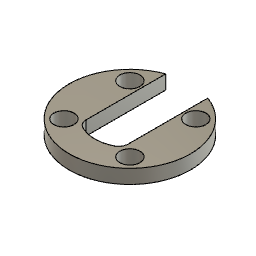
cryo boom 2 v16 (Autodesk Fusion 360 archive; units mm, degrees)
design "cryo clamp lower"
Autodesk Fusion 360 part; units mm, degrees
note: some values were not read from the file. Set by a fixed rule: the direction of a hole.
sketch "Sketch1" plane through (0, 0, 0) normal (0, 1, 0) x (1, 0, 0)
  circle A0 centre (0, 0) radius 13
  circle A1 centre (0, 0) radius 7.5
  line L0 (-4.5, 12.1963) -> (-4.5, -6)
  line L1 (4.5, -6) -> (4.5, 12.1963)
  circle A2 centre (0, 0) radius 10 construction
  line L2 (0, 0) -> (7.0711, -7.0711)
  line L3 (0, 0) -> (13, 0) construction
  point P0 (7.0711, -7.0711)
  dimension "d1" = 26
  dimension "d2" = 15
  dimension "d3" = 9
  dimension "d4" = 20
  dimension "d12" = 45
  constraint coincident A0.centre A1.centre
  constraint coincident A0 L0.start
  constraint coincident A1 L0.end
  constraint vertical L0
  constraint coincident A1 L1.start
  constraint coincident A0 L1.end
  constraint parallel L0 L1
  constraint horizontal L0.end L1.start
  constraint concentric A1 A2
  constraint coincident A2 P0
  constraint coincident P0 L2.end
  constraint coincident A0 L3.end
  constraint perpendicular L1 L3
  measures "d1" diameter of A0
  measures "d2" diameter of A1
  measures "d3" distance of L0 L1
  measures "d4" diameter of A2
  measures "d12" angle of L2 L3
extrude "Extrude1" add sketch "Sketch1" along normal blind 3 contours A0 A1 L0 L1 | A1 L1 L2 | A1 L0 | A1 L1 L2 picked at (8.8444, -6.7794)
hole "Hole1" at (7.0711, 0, 7.0711) direction (0, 1, 0) diameter 4.3 end through all
pattern_circular "C-Pattern1" count 4 over 360 about axis through (0, 1.75, 0) along (0, 1, 0) of "Hole1"
fillet "Fillet1" radius 2 2 edges at (-4.5, 1.5, 6) (4.5, 1.5, 6)
sketch "Sketch2" plane through (0, 3, 0) normal (0, 1, 0) x (-1, 0, 0)
  circle A0 centre (7.0711, 7.0711) radius 2.15
  circle A1 centre (7.0711, -7.0711) radius 2.15
  circle A2 centre (-7.0711, -7.0711) radius 2.15
  circle A3 centre (-7.0711, 7.0711) radius 2.15
  arc A4 (4.5, -12.1963) -> (-4.5, -12.1963) centre (0, 0) ccw
  line L0 (-4.5, -12.1963) -> (-4.5, 4.899)
  arc A5 (-3.4091, 6.6804) -> (-4.5, 4.899) centre (-2.5, 4.899) ccw
  arc A6 (3.4091, 6.6804) -> (-3.4091, 6.6804) centre (0, 0) ccw
  arc A7 (4.5, 4.899) -> (3.4091, 6.6804) centre (2.5, 4.899) ccw
  line L1 (4.5, 4.899) -> (4.5, -12.1963)

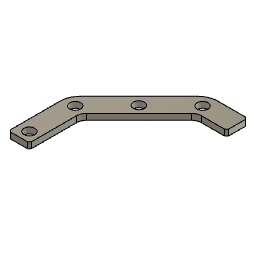
design "stage 2 shield 2 clamps top"
Autodesk Fusion 360 part; units mm, degrees
sketch "Sketch1" plane through (0, 0, 0) normal (0, 1, 0) x (1, 0, 0)
  circle A0 centre (0, 0) radius 55 construction
  line L0 (48, 0) -> (48, 19.8823)
  line L1 (48, 19.8823) -> (19.8823, 48)
  line L2 (19.8823, 48) -> (-19.8823, 48)
  line L3 (-19.8823, 48) -> (-48, 19.8823)
  line L4 (-48, 19.8823) -> (-48, 0)
  line L5 (-48, 0) -> (48, 0) construction
  line L6 (0, -1.75) -> (0, -22.5) construction
  line L7 (50, 0) -> (50, 20.7107)
  line L8 (50, 20.7107) -> (20.7107, 50)
  line L9 (20.7107, 50) -> (-20.7107, 50)
  line L10 (-20.7107, 50) -> (-50, 20.7107)
  line L11 (-50, 20.7107) -> (-50, 0)
  line L12 (0, 0) -> (-54.6194, 22.6241) construction
  line L13 (60.5, 0) -> (60.5, 25.0599)
  line L14 (60.5, 25.0599) -> (25.0599, 60.5)
  line L15 (25.0599, 60.5) -> (-25.0599, 60.5)
  line L16 (-25.0599, 60.5) -> (-60.5, 25.0599)
  line L17 (-60.5, 25.0599) -> (-60.5, 0)
  line L18 (0, 60.5) -> (0, 50)
  line L19 (-50, 0) -> (-50, -5)
  line L20 (-50, -5) -> (-60.5, -5)
  line L21 (-60.5, -5) -> (-60.5, 0)
  line L22 (-6, 60.5) -> (-6, 50)
  point P0 (-55, 0)
  point P1 (-38.8909, -38.8909)
  point P2 (-54.6194, -22.6241)
  point P3 (0, -55)
  point P4 (-22.6241, -54.6194)
  point P5 (38.8909, -38.8909)
  point P6 (22.6241, -54.6194)
  point P7 (55, 0)
  point P8 (54.6194, -22.6241)
  point P9 (38.8909, 38.8909)
  point P10 (54.6194, 22.6241)
  point P11 (0, 55)
  point P12 (22.6241, 54.6194)
  point P13 (-38.8909, 38.8909)
  point P14 (-22.6241, 54.6194)
  dimension "d1" = 110
  dimension "d21" = 96
  dimension "d22" = 48
  dimension "d23" = 45
  dimension "d26" = 2
  dimension "d28" = 5
  dimension "d29" = 12.5
  dimension "d31" = 360
  dimension "d39" = 5
  dimension "d40" = 6
  constraint coincident A0.centre L12.start
  constraint horizontal L2
  constraint coincident A0 P0
  constraint horizontal A0.centre P0
  constraint equal L2 L3
  constraint equal L1 L2
  constraint equal L0 L4
  constraint horizontal L5
  constraint coincident A0.centre L5
  constraint coincident L3.end L12
  constraint coincident L15 L18.start
  constraint coincident L9 L18.end
  constraint perpendicular L9 L18
  constraint coincident P11 L18
  constraint parallel L11 L19
  constraint perpendicular L19 L20
  constraint collinear L17 L21
  measures "d1" diameter of A0
  measures "d21" distance of L0 L4
  measures "d22" distance of A0.centre L2
  measures "d23" angle of L2 L3
  measures "d28" distance of L10.end L12.end
  measures "d39" distance of P0 L20
extrude "Extrude3" add sketch "Sketch1" along normal blind 3 contours L9 L10 L11 L15 L16 L17 L19 L20 L21 L22
hole "Hole2" at (-54.6194, 0, -22.6241) at (-38.8909, 0, -38.8909) at (-22.6241, 0, -54.6194) at (-55, 0, 0) direction (0, 1, 0) diameter 5.5 depth 5 tip angle 118
fillet "Fillet1" radius 10 2 edges at (-60.5, 1.5, -25.0599) (-25.0599, 1.5, -60.5)
fillet "Fillet2" radius 5 2 edges at (-50, 1.5, -20.7107) (-20.7107, 1.5, -50)
chamfer "Chamfer2" distance 1 angle 45 4 edges at (-50, 1.5, 5) (-60.5, 1.5, 5) (-6, 1.5, -50) (-6, 1.5, -60.5)
sketch "Sketch2" plane through (0, 3, 0) normal (0, 1, 0) x (-1, 0, 0)
  line L0 (6, -59.5) -> (7, -60.5)
  line L1 (7, -60.5) -> (20.9178, -60.5)
  arc A0 (20.9178, -60.5) -> (27.9889, -57.5711) centre (20.9178, -50.5) ccw
  line L2 (27.9889, -57.5711) -> (57.5711, -27.9889)
  arc A1 (57.5711, -27.9889) -> (60.5, -20.9178) centre (50.5, -20.9178) ccw
  line L3 (60.5, -20.9178) -> (60.5, 4)
  line L4 (60.5, 4) -> (59.5, 5)
  line L5 (59.5, 5) -> (51, 5)
  line L6 (51, 5) -> (50, 4)
  line L7 (50, 4) -> (50, -18.6396)
  arc A2 (48.5355, -22.1751) -> (50, -18.6396) centre (45, -18.6396) ccw
  line L8 (48.5355, -22.1751) -> (22.1751, -48.5355)
  arc A3 (18.6396, -50) -> (22.1751, -48.5355) centre (18.6396, -45) ccw
  line L9 (18.6396, -50) -> (7, -50)
  line L10 (7, -50) -> (6, -51)
  line L11 (6, -51) -> (6, -59.5)
  circle A4 centre (22.6241, -54.6194) radius 2.75
  circle A5 centre (54.6194, -22.6241) radius 2.75
  circle A6 centre (38.8909, -38.8909) radius 2.75
  circle A7 centre (55, 0) radius 2.75

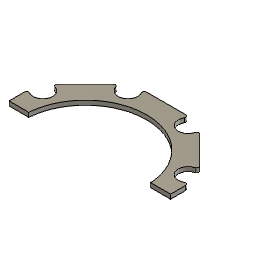
design "stage 1 shield pressure clamp"
Autodesk Fusion 360 part; units mm, degrees
sketch "Sketch1" plane through (0, 0, 0) normal (0, 1, 0) x (1, 0, 0)
  circle A0 centre (0, 0) radius 18 construction
  circle A1 centre (0, 0) radius 14
  circle A2 centre (-16.6298, 6.8883) radius 2.25
  circle A3 centre (-16.6298, -6.8883) radius 2.25
  circle A4 centre (-6.8883, -16.6298) radius 2.25
  circle A5 centre (6.8883, -16.6298) radius 2.25
  circle A6 centre (16.6298, -6.8883) radius 2.25
  circle A7 centre (16.6298, 6.8883) radius 2.25
  circle A8 centre (6.8883, 16.6298) radius 2.25
  circle A9 centre (-6.8883, 16.6298) radius 2.25
  line L0 (-18.5, 7.663) -> (-18.5, -7.663)
  line L1 (-18.5, -7.663) -> (-7.663, -18.5)
  line L2 (-7.663, -18.5) -> (7.663, -18.5)
  line L3 (7.663, -18.5) -> (18.5, -7.663)
  line L4 (18.5, -7.663) -> (18.5, 7.663)
  line L5 (18.5, 7.663) -> (7.663, 18.5)
  line L6 (7.663, 18.5) -> (-7.663, 18.5)
  line L7 (-7.663, 18.5) -> (-18.5, 7.663)
  line L8 (-18.5, 1) -> (18.5, 1)
  point P0 (-16.6298, 6.8883)
  dimension "d1" = 36
  dimension "d2" = 28
  dimension "d3" = 4.5
  dimension "d5" = 360
  dimension "d6" = 18.5
  dimension "d7" = 1
  constraint coincident A0.centre A1.centre
  constraint concentric A0 A1
  constraint coincident A0 P0
  constraint coincident P0 A2.centre
  constraint horizontal A8.centre A9.centre
  constraint horizontal L6
  constraint coincident L0 L8.start
  constraint coincident L4 L8.end
  constraint perpendicular L4 L8
  measures "d1" diameter of A0
  measures "d2" diameter of A1
  measures "d3" diameter of A2
  measures "d6" distance of A0.centre L7
  measures "d7" distance of A0.centre L8
extrude "Extrude1" add sketch "Sketch1" along normal blind 1 contours A1 A2 A7 A8 A9 L0 L4 L5 L6 L7 L8
fillet "Fillet1" radius 0.5 8 edges at (18.5, 0.5, -5.6373) (17.0677, 0.5, -9.0953) (9.0953, 0.5, -17.0677) (5.6373, 0.5, -18.5) (-5.6373, 0.5, -18.5) (-9.0953, 0.5, -17.0677) (-17.0677, 0.5, -9.0953) (-18.5, 0.5, -5.6373)

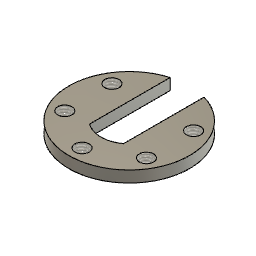
design "cryo clamp upper"
Autodesk Fusion 360 part; units mm, degrees
sketch "Sketch1" plane through (0, 0, 0) normal (0, 1, 0) x (1, 0, 0)
  circle A0 centre (0, 0) radius 16
  circle A1 centre (0, 0) radius 7.5
  line L0 (-4.5, 15.3542) -> (-4.5, -6)
  line L1 (4.5, -6) -> (4.5, 15.3542)
  circle A2 centre (0, 0) radius 12.5 construction
  point P0 (0, -12.5)
  dimension "d1" = 32
  dimension "d2" = 15
  dimension "d3" = 9
  dimension "d4" = 25
  constraint coincident A0.centre A1.centre
  constraint coincident A0 L0.start
  constraint coincident A1 L0.end
  constraint vertical L0
  constraint coincident A1 L1.start
  constraint coincident A0 L1.end
  constraint parallel L0 L1
  constraint horizontal L0.end L1.start
  constraint concentric A1 A2
  constraint coincident A2 P0
  constraint vertical A0.centre P0
  measures "d1" diameter of A0
  measures "d2" diameter of A1
  measures "d3" distance of L0 L1
  measures "d4" diameter of A2
extrude "Extrude1" add sketch "Sketch1" along normal blind 3 contours A0 A1 L0 L1 | A1 L1 | A1 L0 picked at (10.3483, -8.0939) makes body 1
hole "Hole1" at (0, 0, 12.5) direction (0, 1, 0) diameter 3.783 end through all bodies 1
thread "Thread2" "ISO Metric profile 4.5 M4.5x0.75 6H"
pattern_circular "C-Pattern1" count 6 over 360 about axis through (0, 1.75, 0) along (0, 1, 0) of "Hole1"
extrude "Extrude2" add sketch "Sketch1" along normal blind 3 separate body makes body 2
hole "Hole2" at (0, 0, 12.5) direction (0, 1, 0) diameter 4.5 depth 3 tip angle 118 bodies 2
pattern_circular "C-Pattern2" count 6 over 360 about axis through (0, 1.75, 0) along (0, 1, 0) of "Hole2"
hole "Hole3" at (0, 0, 0) direction (0, 1, 0) diameter 2 end through all bodies 2
copy_body "Body->Comp1" bodies 1 removing the originals makes body 3 in component "LC"
copy_body "Body->Comp2" bodies 2 removing the originals makes body 4 in component "UC"
sketch "Sketch2" plane through (0, 3, 0) normal (0, 1, 0) x (-1, 0, 0)
  circle A0 centre (0, 0) radius 1
  circle A1 centre (10.8253, 6.25) radius 2.25
  circle A2 centre (10.8253, -6.25) radius 2.25
  circle A3 centre (0, -12.5) radius 2.25
  circle A4 centre (-10.8253, -6.25) radius 2.25
  circle A5 centre (-10.8253, 6.25) radius 2.25
  circle A6 centre (0, 12.5) radius 2.25
  circle A7 centre (0, 0) radius 16
sketch "Sketch3" plane through (0, 3, 0) normal (0, 1, 0) x (-1, 0, 0)
  circle A0 centre (10.8253, 6.25) radius 1.8916
  circle A1 centre (10.8253, -6.25) radius 1.8916
  circle A2 centre (-10.8253, -6.25) radius 1.8915
  circle A3 centre (-10.8253, 6.25) radius 1.8915
  circle A4 centre (0, 12.5) radius 1.8916
  arc A5 (4.5, -15.3542) -> (-4.5, -15.3542) centre (0, 0) ccw
  line L0 (-4.5, -15.3542) -> (-4.5, 6)
  arc A6 (4.5, 6) -> (-4.5, 6) centre (0, 0) ccw
  line L1 (4.5, 6) -> (4.5, -15.3542)
component "LC" placed x (1, 0, 0) y (0, 1, 0) z (0, 0, 1) at (0, 0, 0)
component "UC" placed x (1, 0, 0) y (0, 1, 0) z (0, 0, 1) at (0, 0, 0)
named bodies: "LC", "UC"

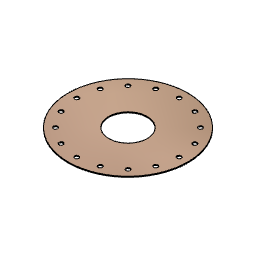
design "shield connector"
Autodesk Fusion 360 part; units mm, degrees
sketch "Sketch1" plane through (0, 0, 0) normal (0, 1, 0) x (1, 0, 0)
  circle A0 centre (0, 0) radius 60 construction
  circle A1 centre (0, 0) radius 22.5
  circle A2 centre (0, 0) radius 70
  point P0 (-60, 0)
  dimension "d1" = 120
  dimension "d2" = 45
  dimension "d3" = 140
  constraint coincident A0.centre A1.centre
  constraint concentric A0 A1
  constraint coincident A0 P0
  constraint horizontal A0.centre P0
  measures "d1" diameter of A0
  measures "d2" diameter of A1
  measures "d3" diameter of A2
extrude "Extrude1" add sketch "Sketch1" along normal blind 1
hole "Hole1" at (-60, 0, 0) direction (0, 1, 0) diameter 5 depth 30 tip angle 118
pattern_circular "C-Pattern1" count 16 over 360 about axis through (0, 1.75, 0) along (0, 1, 0) of "Hole1"
sketch "cutting pattern" plane through (0, 1, 0) normal (0, 1, 0) x (-1, 0, 0)
  circle A0 centre (55.4328, -22.961) radius 2.5
  circle A1 centre (42.4264, -42.4264) radius 2.5
  circle A2 centre (22.961, -55.4328) radius 2.5
  circle A3 centre (0, -60) radius 2.5
  circle A4 centre (-22.961, -55.4328) radius 2.5
  circle A5 centre (-42.4264, -42.4264) radius 2.5
  circle A6 centre (-55.4328, -22.961) radius 2.5
  circle A7 centre (-60, 0) radius 2.5
  circle A8 centre (-55.4328, 22.961) radius 2.5
  circle A9 centre (-42.4264, 42.4264) radius 2.5
  circle A10 centre (-22.961, 55.4328) radius 2.5
  circle A11 centre (0, 60) radius 2.5
  circle A12 centre (22.961, 55.4328) radius 2.5
  circle A13 centre (42.4264, 42.4264) radius 2.5
  circle A14 centre (55.4328, 22.961) radius 2.5
  circle A15 centre (60, 0) radius 2.5
  circle A16 centre (0, 0) radius 22.5
  circle A17 centre (0, 0) radius 70

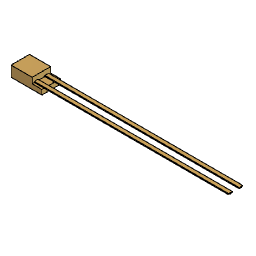
design "Lakeshore DT 670 SD Omega CY 670 SD"
Autodesk Fusion 360 part; units mm, degrees
sketch "Sketch1" plane through (0, 0, 0) normal (0, 0, 1) x (1, 0, 0)
  line L0 (0, 0) -> (3.175, 0)
  line L1 (3.175, 0) -> (3.175, 0.5)
  line L2 (3.175, 0.5) -> (2.175, 0.5)
  line L3 (2.175, 0.5) -> (2.175, 1.08)
  line L4 (2.175, 1.08) -> (0, 1.08)
  line L5 (0, 1.08) -> (0, 0)
  dimension "d1" = 1.08
  dimension "d2" = 3.175
  dimension "d3" = 1
  dimension "d4" = 0.5
  constraint coincident L0.start L5.end
  constraint horizontal L0
  constraint perpendicular L0 L1
  constraint perpendicular L1 L2
  constraint perpendicular L0 L3
  constraint perpendicular L3 L4
  constraint perpendicular L0 L5
  measures "d1" distance of L4.end L0.start
  measures "d2" distance of L0.start L0.end
  measures "d3" distance of L1.end L2.end
  measures "d4" distance of L0.end L1.end
extrude "Extrude1" add sketch "Sketch1" along normal blind 1.905
sketch "Sketch2" plane through (0, 0.5, 0) normal (0, 1, 0) x (-1, 0, 0)
  line L0 (-3.175, 0) -> (-2.175, 0)
  line L1 (-2.175, 0) -> (-2.175, 1.905)
  line L2 (-2.175, 1.905) -> (-3.175, 1.905)
  line L3 (-3.175, 1.905) -> (-3.175, 0)
  line L4 (-2.175, 0.2225) -> (-22.175, 0.2225)
  line L5 (-22.175, 0.2225) -> (-22.175, 0.6035)
  line L6 (-22.175, 0.6035) -> (-2.175, 0.6035)
  line L7 (-2.175, 0.6035) -> (-2.175, 0.2225)
  line L8 (-3.175, 0.9525) -> (0, 0.9525) construction
  line L9 (-2.175, 1.6825) -> (-22.175, 1.6825)
  line L10 (-22.175, 1.3015) -> (-2.175, 1.3015)
  line L11 (-22.175, 1.6825) -> (-22.175, 1.3015)
  line L12 (-2.175, 1.3015) -> (-2.175, 1.6825)
  dimension "d7" = 0.381
  dimension "d8" = 19
  dimension "d9" = 0.698
  constraint horizontal L4
  constraint vertical L5
  constraint horizontal L6
  constraint vertical L7
  constraint collinear L1 L7
  constraint midpoint L3 L8.start
  constraint perpendicular L3 L8
  constraint symmetric L4.start L8 L9.start
  constraint symmetric L4.end L8 L9.end
  constraint symmetric L5.end L8 L10.start
  constraint symmetric L6.end L8 L10.end
  measures "d7" distance of L4.end L5.end
  measures "d8" distance of L3 L5
  measures "d9" distance of L6 L10
extrude "Extrude2" add sketch "Sketch2" along normal blind 0.102 contours L3 L4 L5 L6 | L1 L3 L4 L6 L7 | L3 L9 L10 L11 | L1 L3 L9 L10 L12

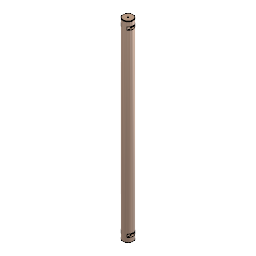
design "thermal conductor"
Autodesk Fusion 360 part; units mm, degrees
sketch "Sketch1" plane through (0, 0, 0) normal (0, 0, 1) x (1, 0, 0)
  line L0 (-7.5, 0) -> (7.5, 0)
  line L1 (7.5, 0) -> (7.5, 275)
  line L2 (7.5, 275) -> (-7.5, 275)
  line L3 (-7.5, 275) -> (-7.5, 0)
  line L4 (-7.5, 7) -> (-4.5, 7)
  line L5 (-4.5, 7) -> (-4.5, 11)
  line L6 (-4.5, 11) -> (-7.5, 11)
  line L7 (0, 0) -> (0, 275)
  dimension "d1" = 15
  dimension "d2" = 275
  dimension "d3" = 7
  dimension "d4" = 4
  dimension "d5" = 3
  constraint horizontal L0
  constraint perpendicular L0 L1
  constraint perpendicular L1 L2
  constraint perpendicular L0 L3
  constraint midpoint L7.start L0
  constraint coincident L3 L4.start
  constraint perpendicular L3 L4
  constraint perpendicular L4 L5
  constraint coincident L3 L6.end
  constraint perpendicular L3 L6
  constraint coincident L7.start origin
  constraint midpoint L2 L7.end
  measures "d1" distance of L1 L3
  measures "d2" distance of L0.end L1.end
  measures "d3" distance of L0 L4
  measures "d4" distance of L4.end L5.end
  measures "d5" distance of L3 L5
revolve "Revolve1" add sketch "Sketch1" angle 360 about axis through (0, 0, 0) along (0, 1, 0) contours L0 L1 L2 L7
extrude "Extrude1" cut sketch "Sketch1" along normal through all and the other way through all contours L3 L4 L5 L6
mirror "Mirror1" about plane through (0, 0, 0) normal (1, 0, 0) of "Extrude1"
ref_plane "WorkPlane1" through (0, 137.5, 0) normal (0, -1, 0) x (0, 0, -1)
hole "Hole2" at (0, 0, 0) direction (0, 1, 0) diameter 1.5 depth 5 tip angle 118
mirror "Mirror2" about plane through (0, 137.5, 0) normal (0, -1, 0) of "Extrude1", "Mirror1", "Hole2"
chamfer "Chamfer1" distance 0.5 angle 45 2 edges at (-6.9925, 0, -2.7121) (-6.9925, 275, -2.7121)

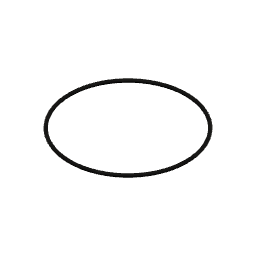
design "O ring 145 x 4"
Autodesk Fusion 360 part; units mm, degrees
sketch "Sketch1" plane through (0, 0, 0) normal (0, 0, 1) x (1, 0, 0)
  circle A0 centre (74.5, 0) radius 2
  dimension "d1" = 4
  dimension "d2" = 74.5
  constraint horizontal origin A0.centre
  measures "d1" diameter of A0
  measures "d2" horizontal distance of origin A0.centre
revolve "Revolve1" add sketch "Sketch1" angle 360 about axis through (0, 1.75, 0) along (0, 1, 0)
equation "d2 = ( 145 / 2 ) * 1 mm + 2 mm"

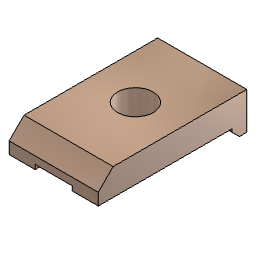
design "CY7 diode clamp"
Autodesk Fusion 360 part; units mm, degrees
sketch "Sketch1" plane through (0, 0, 0) normal (0, 1, 0) x (1, 0, 0)
  line L0 (-3, 4.5) -> (3, 4.5)
  line L1 (3, 4.5) -> (3, -5.5)
  line L2 (3, -5.5) -> (-3, -5.5)
  line L3 (-3, -5.5) -> (-3, 4.5)
  line L4 (-1.25, -5.5) -> (-1.25, -2.5)
  arc A0 (1.25, -2.5) -> (-1.25, -2.5) centre (0, -2.5) ccw
  line L5 (1.25, -2.5) -> (1.25, -5.5)
  line L6 (-3, 3.5) -> (3, 3.5)
  line L7 (0, 0) -> (0, -2.5) construction
  dimension "d2" = 2.5
  dimension "d3" = 3
  dimension "d4" = 1
  dimension "d5" = 10
  dimension "d6" = 2.5
  dimension "d7" = 6
  constraint horizontal L0
  constraint vertical L1
  constraint horizontal L2
  constraint vertical L3
  constraint coincident L2 L4.start
  constraint perpendicular L2 L4
  constraint tangent L4 A0
  constraint coincident L2 L5.end
  constraint tangent A0 L5
  constraint perpendicular L2 L5
  constraint coincident L3 L6.start
  constraint coincident L1 L6.end
  constraint perpendicular L1 L6
  constraint coincident L7.start origin
  constraint vertical L7.start A0.centre
  constraint coincident A0.centre L7.end
  constraint symmetric L1 L3 L7
  measures "d2" distance of L4 L5
  measures "d3" distance of L2 A0.centre
  measures "d4" distance of L0 L6
  measures "d5" distance of L0 L2
  measures "d6" distance of A0.centre L7.start
  measures "d7" distance of L1 L3
extrude "Extrude1" add sketch "Sketch1" along normal blind 2.5
extrude "Extrude2" cut sketch "Sketch1" along normal blind 0.7 contours L1 L2 L3 L4 A0 L5 L6 | L2 L4 A0 L5
extrude "Extrude3" cut sketch "Sketch1" along normal blind 1 contours L2 L4 A0 L5
hole "Hole1" at (0, 0, 0) direction (0, 1, 0) diameter 2.4 depth 5 tip angle 118
chamfer "Chamfer1" distance 0.5 angle 45 1 edges at (0, 0, -3.5)
chamfer "Chamfer2" distance 1 angle 45 1 edges at (0, 2.5, 5.5)

design "cryo contact clamp"
Autodesk Fusion 360 part; units mm, degrees
sketch "Sketch1" plane through (0, 0, 0) normal (0, 0, 1) x (1, 0, 0)
  circle A0 centre (0, 0) radius 10 construction
  circle A1 centre (0, 0) radius 13
  point P0 (10, 0)
  point P1 (0, 10)
  point P2 (-10, 0)
  point P3 (0, -10)
  dimension "d1" = 20
  dimension "d2" = 26
  dimension "d4" = 360
  constraint coincident A0.centre A1.centre
  constraint coincident A0 P0
  constraint horizontal A0.centre P0
  measures "d1" diameter of A0
  measures "d2" diameter of A1
extrude "Extrude1" add sketch "Sketch1" along normal blind 2
hole "Hole1" at (-10, 0, 0) at (0, -10, 0) at (10, 0, 0) at (0, 10, 0) direction (0, 0, 1) diameter 4.8 depth 10 tip angle 118
chamfer "Chamfer1" distance 1 angle 45 1 edges at (-12.1203, -4.701, 2)

design "stage 2 connector clamp"
Autodesk Fusion 360 part; units mm, degrees
sketch "Sketch1" plane through (0, 0, 0) normal (0, 1, 0) x (1, 0, 0)
  circle A0 centre (0, 0) radius 60 construction
  line L0 (-65, -26.9239) -> (-26.9239, -65)
  line L1 (-26.9239, -65) -> (26.9239, -65)
  line L2 (26.9239, -65) -> (65, -26.9239)
  line L3 (65, -26.9239) -> (65, 26.9239)
  line L4 (65, 26.9239) -> (26.9239, 65)
  line L5 (26.9239, 65) -> (-26.9239, 65)
  line L6 (-26.9239, 65) -> (-65, 26.9239)
  line L7 (-65, 26.9239) -> (-65, -26.9239)
  line L8 (-20.7107, -50) -> (20.7107, -50)
  line L9 (20.7107, -50) -> (50, -20.7107)
  line L10 (50, -20.7107) -> (50, 20.7107)
  line L11 (50, 20.7107) -> (20.7107, 50)
  line L12 (20.7107, 50) -> (-20.7107, 50)
  line L13 (-20.7107, 50) -> (-50, 20.7107)
  line L14 (-50, 20.7107) -> (-50, -20.7107)
  line L15 (-50, -20.7107) -> (-20.7107, -50)
  point P0 (-60, 0)
  dimension "d1" = 120
  dimension "d2" = 65
  dimension "d3" = 130
  dimension "d4" = -15
  constraint coincident A0.centre origin
  constraint coincident A0 P0
  constraint horizontal A0.centre P0
  constraint horizontal L5
  measures "d1" diameter of A0
  measures "d2" distance of A0.centre L7
  measures "d3" distance of L3 L7 A0.centre
extrude "Extrude1" add sketch "Sketch1" along normal blind 2.5
hole "Hole1" at (-60, 0, 0) direction (0, 1, 0) diameter 4.234 depth 100 tip angle 118
thread "Thread1" "ISO Metric profile 5.0 M5x0.8 6H"
pattern_circular "C-Pattern1" count 16 over 360 about axis through (0, 1.75, 0) along (0, 1, 0) of "Hole1"
fillet "Fillet1" radius 8 16 edges at (-26.9239, 1.25, 65) (26.9239, 1.25, 65) (65, 1.25, 26.9239) (65, 1.25, -26.9239) (26.9239, 1.25, -65) (-26.9239, 1.25, -65) (-65, 1.25, -26.9239) (-65, 1.25, 26.9239) (20.7107, 1.25, -50) (50, 1.25, -20.7107) (50, 1.25, 20.7107) (20.7107, 1.25, 50) (-20.7107, 1.25, 50) (-50, 1.25, 20.7107) (-50, 1.25, -20.7107) (-20.7107, 1.25, -50)
sketch "stage 2 connector clamp cutting pattern" plane through (0, 2.5, 0) normal (0, 1, 0) x (-1, 0, 0)
  arc A0 (65, 23.6102) -> (62.6569, 29.267) centre (57, 23.6102) ccw
  line L0 (62.6569, 29.267) -> (29.267, 62.6569)
  arc A1 (29.267, 62.6569) -> (23.6102, 65) centre (23.6102, 57) ccw
  line L1 (23.6102, 65) -> (-23.6102, 65)
  arc A2 (-23.6102, 65) -> (-29.267, 62.6569) centre (-23.6102, 57) ccw
  line L2 (-29.267, 62.6569) -> (-62.6569, 29.267)
  arc A3 (-62.6569, 29.267) -> (-65, 23.6102) centre (-57, 23.6102) ccw
  line L3 (-65, 23.6102) -> (-65, -23.6102)
  arc A4 (-65, -23.6102) -> (-62.6569, -29.267) centre (-57, -23.6102) ccw
  line L4 (-62.6569, -29.267) -> (-29.267, -62.6569)
  arc A5 (-29.267, -62.6569) -> (-23.6102, -65) centre (-23.6102, -57) ccw
  line L5 (-23.6102, -65) -> (23.6102, -65)
  arc A6 (23.6102, -65) -> (29.267, -62.6569) centre (23.6102, -57) ccw
  line L6 (29.267, -62.6569) -> (62.6569, -29.267)
  arc A7 (62.6569, -29.267) -> (65, -23.6102) centre (57, -23.6102) ccw
  line L7 (65, -23.6102) -> (65, 23.6102)
  circle A8 centre (55.4328, -22.961) radius 2.117
  circle A9 centre (42.4264, -42.4264) radius 2.117
  circle A10 centre (22.961, -55.4328) radius 2.117
  circle A11 centre (0, -60) radius 2.117
  circle A12 centre (-22.961, -55.4328) radius 2.117
  circle A13 centre (-42.4264, -42.4264) radius 2.117
  circle A14 centre (-55.4328, -22.961) radius 2.117
  circle A15 centre (-60, 0) radius 2.117
  circle A16 centre (-55.4328, 22.961) radius 2.117
  circle A17 centre (-42.4264, 42.4264) radius 2.117
  circle A18 centre (-22.961, 55.4328) radius 2.117
  circle A19 centre (0, 60) radius 2.117
  circle A20 centre (22.961, 55.4328) radius 2.117
  circle A21 centre (42.4264, 42.4264) radius 2.117
  circle A22 centre (55.4328, 22.961) radius 2.117
  circle A23 centre (60, 0) radius 2.117
  line L8 (23.0538, 47.6569) -> (47.6569, 23.0538)
  arc A24 (50, 17.397) -> (47.6569, 23.0538) centre (42, 17.397) ccw
  line L9 (50, 17.397) -> (50, -17.397)
  arc A25 (47.6569, -23.0538) -> (50, -17.397) centre (42, -17.397) ccw
  line L10 (47.6569, -23.0538) -> (23.0538, -47.6569)
  arc A26 (17.397, -50) -> (23.0538, -47.6569) centre (17.397, -42) ccw
  line L11 (17.397, -50) -> (-17.397, -50)
  arc A27 (-23.0538, -47.6569) -> (-17.397, -50) centre (-17.397, -42) ccw
  line L12 (-23.0538, -47.6569) -> (-47.6569, -23.0538)
  arc A28 (-50, -17.397) -> (-47.6569, -23.0538) centre (-42, -17.397) ccw
  line L13 (-50, -17.397) -> (-50, 17.397)
  arc A29 (-47.6569, 23.0538) -> (-50, 17.397) centre (-42, 17.397) ccw
  line L14 (-47.6569, 23.0538) -> (-23.0538, 47.6569)
  arc A30 (-17.397, 50) -> (-23.0538, 47.6569) centre (-17.397, 42) ccw
  line L15 (-17.397, 50) -> (17.397, 50)
  arc A31 (23.0538, 47.6569) -> (17.397, 50) centre (17.397, 42) ccw

design "stage 2 shield 2 clamps"
Autodesk Fusion 360 part; units mm, degrees
sketch "Sketch1" plane through (0, 0, 0) normal (0, 1, 0) x (1, 0, 0)
  circle A0 centre (0, 0) radius 55 construction
  line L0 (48, 0) -> (48, 19.8823)
  line L1 (48, 19.8823) -> (19.8823, 48)
  line L2 (19.8823, 48) -> (-19.8823, 48)
  line L3 (-19.8823, 48) -> (-48, 19.8823)
  line L4 (-48, 19.8823) -> (-48, 0)
  line L5 (-48, 0) -> (48, 0) construction
  line L6 (0, -1.75) -> (0, -22.5) construction
  line L7 (50, 0) -> (50, 20.7107)
  line L8 (50, 20.7107) -> (20.7107, 50)
  line L9 (20.7107, 50) -> (-20.7107, 50)
  line L10 (-20.7107, 50) -> (-50, 20.7107)
  line L11 (-50, 20.7107) -> (-50, 0)
  line L12 (0, 0) -> (-54.6194, 22.6241) construction
  line L13 (60.5, 0) -> (60.5, 25.0599)
  line L14 (60.5, 25.0599) -> (25.0599, 60.5)
  line L15 (25.0599, 60.5) -> (-25.0599, 60.5)
  line L16 (-25.0599, 60.5) -> (-60.5, 25.0599)
  line L17 (-60.5, 25.0599) -> (-60.5, 0)
  line L18 (0, 60.5) -> (0, 50)
  line L19 (-50, 0) -> (-50, -5)
  line L20 (-50, -5) -> (-60.5, -5)
  line L21 (-60.5, -5) -> (-60.5, 0)
  line L22 (-6, 60.5) -> (-6, 50)
  point P0 (-55, 0)
  point P1 (-38.8909, -38.8909)
  point P2 (-54.6194, -22.6241)
  point P3 (0, -55)
  point P4 (-22.6241, -54.6194)
  point P5 (38.8909, -38.8909)
  point P6 (22.6241, -54.6194)
  point P7 (55, 0)
  point P8 (54.6194, -22.6241)
  point P9 (38.8909, 38.8909)
  point P10 (54.6194, 22.6241)
  point P11 (0, 55)
  point P12 (22.6241, 54.6194)
  point P13 (-38.8909, 38.8909)
  point P14 (-22.6241, 54.6194)
  dimension "d1" = 110
  dimension "d21" = 96
  dimension "d22" = 48
  dimension "d23" = 45
  dimension "d26" = 2
  dimension "d28" = 5
  dimension "d29" = 12.5
  dimension "d31" = 360
  dimension "d39" = 5
  dimension "d40" = 6
  constraint coincident A0.centre L12.start
  constraint horizontal L2
  constraint coincident A0 P0
  constraint horizontal A0.centre P0
  constraint equal L2 L3
  constraint equal L1 L2
  constraint equal L0 L4
  constraint horizontal L5
  constraint coincident A0.centre L5
  constraint coincident L3.end L12
  constraint coincident L15 L18.start
  constraint coincident L9 L18.end
  constraint perpendicular L9 L18
  constraint coincident P11 L18
  constraint parallel L11 L19
  constraint perpendicular L19 L20
  constraint collinear L17 L21
  measures "d1" diameter of A0
  measures "d21" distance of L0 L4
  measures "d22" distance of A0.centre L2
  measures "d23" angle of L2 L3
  measures "d28" distance of L10.end L12.end
  measures "d39" distance of P0 L20
extrude "Extrude3" add sketch "Sketch1" along normal blind 2.5 contours L9 L10 L11 L15 L16 L17 L19 L20 L21 L22
hole "Hole2" at (-54.6194, 0, -22.6241) at (-38.8909, 0, -38.8909) at (-22.6241, 0, -54.6194) at (-55, 0, 0) direction (0, 1, 0) diameter 4.234 depth 5 tip angle 118
thread "Thread1" "ISO Metric profile 5.0 M5x0.8 6H"
fillet "Fillet1" radius 10 2 edges at (-60.5, 1.25, -25.0599) (-25.0599, 1.25, -60.5)
fillet "Fillet2" radius 5 2 edges at (-50, 1.25, -20.7107) (-20.7107, 1.25, -50)
chamfer "Chamfer2" distance 1 angle 45 4 edges at (-50, 1.25, 5) (-60.5, 1.25, 5) (-6, 1.25, -50) (-6, 1.25, -60.5)
sketch "stage 2 shield clamps cutting pattern" plane through (0, 2.5, 0) normal (0, 1, 0) x (-1, 0, 0)
  line L0 (6, -59.5) -> (7, -60.5)
  line L1 (7, -60.5) -> (20.9178, -60.5)
  arc A0 (20.9178, -60.5) -> (27.9889, -57.5711) centre (20.9178, -50.5) ccw
  line L2 (27.9889, -57.5711) -> (57.5711, -27.9889)
  arc A1 (57.5711, -27.9889) -> (60.5, -20.9178) centre (50.5, -20.9178) ccw
  line L3 (60.5, -20.9178) -> (60.5, 4)
  line L4 (60.5, 4) -> (59.5, 5)
  line L5 (59.5, 5) -> (51, 5)
  line L6 (51, 5) -> (50, 4)
  line L7 (50, 4) -> (50, -18.6396)
  arc A2 (48.5355, -22.1751) -> (50, -18.6396) centre (45, -18.6396) ccw
  line L8 (48.5355, -22.1751) -> (22.1751, -48.5355)
  arc A3 (18.6396, -50) -> (22.1751, -48.5355) centre (18.6396, -45) ccw
  line L9 (18.6396, -50) -> (7, -50)
  line L10 (7, -50) -> (6, -51)
  line L11 (6, -51) -> (6, -59.5)
  circle A4 centre (22.6241, -54.6194) radius 2.117
  circle A5 centre (54.6194, -22.6241) radius 2.117
  circle A6 centre (38.8909, -38.8909) radius 2.117
  circle A7 centre (55, 0) radius 2.117

design "Omega CY7 SD7"
Autodesk Fusion 360 part; units mm, degrees
sketch "Sketch1" plane through (0, 0, 0) normal (0, 0, 1) x (1, 0, 0)
  line L0 (0, 0) -> (3.2, 0)
  line L1 (3.2, 0) -> (3.2, 0.5)
  line L2 (3.2, 0.5) -> (2.16, 0.5)
  line L3 (2.16, 0.5) -> (2.16, 0.98)
  line L4 (2.16, 0.98) -> (0, 0.98)
  line L5 (0, 0.98) -> (0, 0)
  dimension "d1" = 3.2
  dimension "d2" = 0.98
  dimension "d3" = 2.16
  dimension "d4" = 0.5
  constraint coincident L0.start L5.end
  constraint horizontal L0
  constraint perpendicular L0 L1
  constraint perpendicular L1 L2
  constraint perpendicular L0 L3
  constraint perpendicular L3 L4
  constraint perpendicular L0 L5
  measures "d1" distance of L0.start L0.end
  measures "d2" distance of L4.end L0.start
  measures "d3" distance of L3.end L4.end
  measures "d4" distance of L0.end L1.end
extrude "Extrude1" add sketch "Sketch1" along normal blind 1.84
sketch "Sketch2" plane through (0, 0.5, 0) normal (0, 1, 0) x (-1, 0, 0)
  line L0 (-3.2, 0) -> (-2.16, 0)
  line L1 (-2.16, 0) -> (-2.16, 1.84)
  line L2 (-2.16, 1.84) -> (-3.2, 1.84)
  line L3 (-3.2, 1.84) -> (-3.2, 0)
  line L4 (-2.16, 0.22) -> (-15.9, 0.22)
  line L5 (-15.9, 0.22) -> (-15.9, 0.6)
  line L6 (-15.9, 0.6) -> (-2.16, 0.6)
  line L7 (-2.16, 0.6) -> (-2.16, 0.22)
  line L8 (-3.2, 0.92) -> (-9.9691, 0.92) construction
  line L9 (-2.16, 1.24) -> (-2.16, 1.62)
  line L10 (-2.16, 1.62) -> (-15.9, 1.62)
  line L11 (-15.9, 1.24) -> (-2.16, 1.24)
  line L12 (-15.9, 1.62) -> (-15.9, 1.24)
  dimension "d7" = 1.4
  dimension "d8" = 0.38
  dimension "d9" = 12.7
  constraint horizontal L4
  constraint vertical L5
  constraint horizontal L6
  constraint vertical L7
  constraint midpoint L3 L8.start
  constraint perpendicular L3 L8
  constraint symmetric L4.start L8 L9.end
  constraint symmetric L4.end L8 L10.end
  constraint symmetric L5.end L8 L11.start
  constraint symmetric L6.end L8 L9.start
  constraint collinear L1 L7
  measures "d7" distance of L4 L10
  measures "d8" distance of L10 L11
  measures "d9" distance of L2.end L12
extrude "Extrude2" add sketch "Sketch2" along normal blind 0.1 contours L3 L4 L5 L6 | L1 L3 L4 L6 L7 | L3 L10 L11 L12 | L1 L3 L9 L10 L11

design "cryo head clamp"
Autodesk Fusion 360 part; units mm, degrees
sketch "Sketch1" plane through (0, 0, 0) normal (0, 1, 0) x (1, 0, 0)
  circle A0 centre (0, 0) radius 29 construction
  circle A1 centre (0, 0) radius 34
  line L0 (32.3381, 10.5) -> (10, 10.5)
  line L1 (10, 10.5) -> (10, -10.5)
  line L2 (10, -10.5) -> (32.3381, -10.5)
  point P0 (0, 29)
  dimension "d1" = 58
  dimension "d2" = 68
  dimension "d3" = 21
  dimension "d4" = 10
  constraint coincident A0.centre A1.centre
  constraint concentric A0 A1
  constraint coincident A1 L0.start
  constraint horizontal L0
  constraint perpendicular L0 L1
  constraint coincident A1 L2.end
  constraint perpendicular L1 L2
  constraint vertical L0.start L2.end
  constraint coincident A0 P0
  constraint vertical A0.centre P0
  measures "d1" diameter of A0
  measures "d2" diameter of A1
  measures "d3" distance of L0 L2
  measures "d4" distance of A0.centre L1
extrude "Extrude1" add sketch "Sketch1" along normal blind 3 contours A1 L0 L1 L2 picked at (-4.6667, 0)
hole "Hole1" at (0, 0, -29) direction (0, 1, 0) diameter 5.8 depth 3 tip angle 118
pattern_circular "C-Pattern1" count 12 over 360 about axis through (0, 1.75, 0) along (0, 1, 0) of "Hole1"
fillet "Fillet1" radius 2 4 edges at (10, 1.5, -10.5) (10, 1.5, 10.5) (32.3381, 1.5, -10.5) (32.3381, 1.5, 10.5)
sketch "Sketch2" plane through (0, 3, 0) normal (0, 1, 0) x (-1, 0, 0)
  circle A0 centre (-14.5, -25.1147) radius 2.9
  circle A1 centre (-14.5, 25.1147) radius 2.9
  circle A2 centre (0, 29) radius 2.9
  circle A3 centre (14.5, 25.1147) radius 2.9
  circle A4 centre (25.1147, 14.5) radius 2.9
  circle A5 centre (29, 0) radius 2.9
  circle A6 centre (25.1147, -14.5) radius 2.9
  circle A7 centre (14.5, -25.1147) radius 2.9
  circle A8 centre (0, -29) radius 2.9
  arc A9 (-31.2987, 13.2812) -> (-29.4576, 10.5) centre (-29.4576, 12.5) ccw
  line L0 (-29.4576, 10.5) -> (-12, 10.5)
  arc A10 (-10, 8.5) -> (-12, 10.5) centre (-12, 8.5) ccw
  line L1 (-10, 8.5) -> (-10, -8.5)
  arc A11 (-12, -10.5) -> (-10, -8.5) centre (-12, -8.5) ccw
  line L2 (-12, -10.5) -> (-29.4576, -10.5)
  arc A12 (-29.4576, -10.5) -> (-31.2987, -13.2813) centre (-29.4576, -12.5) ccw
  arc A13 (-31.2987, -13.2812) -> (-31.2987, 13.2812) centre (0, 0) ccw
  circle A14 centre (-25.1147, -14.5) radius 2.9
  circle A15 centre (-25.1147, 14.5) radius 2.9

design "Lakeshore CO clamp"
Autodesk Fusion 360 part; units mm, degrees
sketch "Sketch1" plane through (0, 0, 0) normal (0, 0, 1) x (1, 0, 0)
  line L0 (0, 0) -> (0, 3.2)
  line L1 (0, 3.2) -> (-7.9, 3.2)
  line L2 (-7.9, 3.2) -> (-7.9, 0.9)
  line L3 (-7.9, 0.9) -> (-1, 0.9)
  line L4 (-1, 0.9) -> (-1, 0)
  line L5 (-1, 0) -> (0, 0)
  dimension "d1" = 3.2
  dimension "d2" = 7.9
  dimension "d3" = 0.9
  dimension "d4" = 1
  constraint coincident L0.start L5.end
  constraint vertical L0
  constraint perpendicular L0 L1
  constraint perpendicular L1 L2
  constraint perpendicular L2 L3
  constraint perpendicular L1 L4
  constraint perpendicular L0 L5
  measures "d1" distance of L0.start L0.end
  measures "d2" distance of L0.end L1.end
  measures "d3" distance of L3.end L4.end
  measures "d4" distance of L4.end L0.start
extrude "Extrude1" add sketch "Sketch1" along normal blind 5.1
hole "Hole1" at (-3.95, 3.2, 2.55) direction (0, -1, 0) diameter 3.264 depth 5 tip angle 118
sketch "Sketch2" plane through (0, 0, 0) normal (0, 1, 0) x (1, 0, 0)
  circle A0 centre (-3.95, -2.55) radius 2
  circle A1 centre (-3.95, -2.55) radius 1.632
  dimension "d10" = 4
  constraint concentric A0 A1
  measures "d10" diameter of A0
extrude "Extrude2" add sketch "Sketch2" along normal up to surface (10.1 mm away) contours A1
